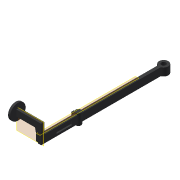
# Autodesk Inventor part: lock
Saved by Autodesk Inventor 2022 Beta2 (Build 260130000, 130) ContinuousBuild 0
## iProperties
Shininess: 64.0
Length Units: 11269
Angle Units: 11279
Time Units: 11290
Mass Units: 11286
Length Display Precision: 3
Angle Display Precision: 2
Created: 2002-04-26
Part Number: lock
Document SubType Name: Modeling
Designer: Administrator
Density: 1 g/cm^3
Material: Generic
Appearance: Generic
Density: 0.0
Volumn: 0.0
Area: 0.0
PropertySet Name: Model Information
Control State: 0
Master: False
Checked Out: False
Author: Administrator
Autodesk Inventor part; units mm, degrees
ref_plane "YZ Plane" through (0, 0, 0) normal (1, 0, 0) x (0, 1, 0)
ref_plane "XZ Plane" through (0, 0, 0) normal (0, 1, 0) x (-1, 0, 0)
ref_plane "XY Plane" through (0, 0, 0) normal (0, 0, 1) x (1, 0, 0)
sketch "Sketch1" plane through (0, 0, 0) normal (0, 0, 1) x (1, 0, 0)
  line L0 (-33.82, 21.26) -> (-13.5, 21.26)
  line L1 (-13.5, 21.26) -> (-13.5, 6.02)
  line L2 (-13.5, 6.02) -> (-16.04, 6.02)
  line L3 (-16.04, 6.02) -> (-18.58, 16.18)
  line L4 (-18.58, 16.18) -> (-33.82, 16.18)
  line L5 (-33.82, 16.18) -> (-33.82, 21.26)
  dimension "d0" = 20.32
  dimension "d1" = 15.24
  dimension "d2" = 5.08
  dimension "d3" = 2.54
  dimension "d4" = 15.24
  constraints: 12 end point, 3 parallel, 1 horizontal, 1 perpendicular
  measures "d0" distance of L0.start L0.end
  measures "d1" distance of L0.end L1.end
  measures "d2" distance of L4.end L0.start
  measures "d3" distance of L1.end L2.end
  measures "d4" distance of L3.end L4.end
extrude "Extrusion1" add sketch "Sketch1" along normal blind 2.54
ref_plane "Work Plane1" through (0, 0, 1.27) normal (0, 0, 1) x (1, 0, 0)
sketch "Sketch2" plane through (0, 0, 1.27) normal (0, 0, 1) x (1, 0, 0)
  line L0 (-33.82, 18.974) -> (-36.36, 18.974)
  arc A0 (-36.36, 18.974) -> (-35.5534, 12.624) centre (-10.96, 18.974) ccw
  line L1 (-35.5534, 12.624) -> (-33.82, 12.624)
  line L2 (-33.82, 12.624) -> (-33.82, 18.974)
  line L3 (-33.82, 16.18) -> (-33.82, 21.26) projected
  line L4 (-33.82, 21.26) -> (-13.5, 21.26) projected
  dimension "d8" = 2.54
  dimension "d9" = 6.35
  dimension "d10" = 25.4
  dimension "d11" = 2.286
  constraints: 6 end point, 2 point on circle, 1 centre point, 1 collinear, 1 horizontal, 1 parallel, 1 perpendicular, 1 point on line
  measures "d8" distance of L0.start L0.end
  measures "d9" distance from line of L0 L1.end
  measures "d10" radius of A0
  measures "d11" distance between parallel lines of L0 L4
revolve "Revolution1" add sketch "Sketch2" angle 360 about axis through (-33.82, 18.974, 1.27) along (-1, 0, 0)
sketch "Sketch3" plane through (0, 0, 1.27) normal (0, 0, 1) x (1, 0, 0)
  line L0 (-16.04, 6.02) -> (-18.58, 6.02)
  line L1 (-18.58, 6.02) -> (-18.58, 18.72)
  line L2 (-18.58, 18.72) -> (-16.04, 18.72)
  line L3 (-16.04, 18.72) -> (-16.04, 6.02)
  line L4 (-13.5, 6.02) -> (-16.04, 6.02) projected
  dimension "d13" = 12.7
  dimension "d14" = 2.54
  constraints: 8 end point, 2 parallel, 1 collinear, 1 horizontal, 1 perpendicular
  measures "d13" distance of L0.end L1.end
  measures "d14" distance of L0.start L0.end
extrude "Extrusion2" add sketch "Sketch3" along normal mid plane 1.016
sketch "Sketch4" plane through (-13.5, 6.02, 0) normal (1, 0, 0) x (0, 0, -1)
  line L0 (-2.54, 15.24) -> (-2.54, 0) projected
  line L1 (0, 15.24) -> (-2.54, 15.24) projected
  line L2 (-2.54, 0) -> (99.06, 0)
  line L3 (-2.54, 6.35) -> (99.06, 6.35)
  line L4 (99.06, 6.35) -> (99.06, 0)
  dimension "d17" = 6.35
  dimension "d18" = 101.6
  constraints: 6 end point, 2 parallel, 1 perpendicular, 1 point on line
  measures "d17" distance of L3.end L2.end
  measures "d18" distance of L0.end L2.end
extrude "Extrusion3" add sketch "Sketch4" against normal blind 2.54
ref_plane "Work Plane2" through (-13.5, 13.64, 0) normal (0, 1, 0) x (1, 0, 0)
sketch "Sketch5" plane through (-13.5, 13.64, 0) normal (0, 1, 0) x (1, 0, 0)
  circle A0 centre (-1.27, 29.21) radius 2.286
  line L0 (0, 99.06) -> (0, 0) projected
  line L1 (-20.32, -2.54) -> (0, -2.54) projected
  dimension "d22" = 4.572
  dimension "d23" = 1.27
  dimension "d24" = 31.75
  constraints: 1 centre point
  measures "d22" diameter of A0
  measures "d23" distance from line of L0 A0.centre
  measures "d24" distance from line of A0.centre L1
extrude "Extrusion4" add sketch "Sketch5" against normal blind 8.89
sketch "Sketch6" plane through (-16.04, 12.37, 0) normal (0, 1, 0) x (1, 0, 0)
  arc A0 (0, 27.3092) -> (2.54, 27.3092) centre (1.27, 29.21) ccw projected
  line L0 (0, 27.3092) -> (0, 0) projected
  line L1 (2.54, 27.3092) -> (2.54, 0) projected
  line L2 (1.27, 29.21) -> (-2.54, 29.21)
  line L3 (-2.54, 29.21) -> (-2.54, 27.178)
  line L4 (-2.54, 27.178) -> (1.27, 27.178)
  line L5 (1.27, 27.178) -> (1.27, 29.21)
  line L6 (-2.54, -1.778) -> (-2.54, -0.762) projected
  dimension "d27" = 2.032
  constraints: 8 end point, 3 perpendicular, 1 collinear, 1 parallel
  measures "d27" distance of L2.end L3.end
extrude "Extrusion5" add sketch "Sketch6" against normal up to surface (6.35 mm away)
sketch "Sketch7" plane through (-16.04, 6.02, -99.06) normal (0, -1, 0) x (1, 0, 0)
  line L0 (0, 67.9492) -> (0, 0) projected
  line L1 (2.54, 67.9492) -> (2.54, 0) projected
  circle A0 centre (1.27, 0) radius 3.81
  circle A1 centre (1.27, 0) radius 1.27 construction
  arc A2 (2.54, 71.7508) -> (-1.016, 69.85) centre (1.27, 69.85) ccw projected
  dimension "d31" = 7.62
  dimension "d42" = 69.85
  constraints: 2 centre point, 2 tangent, 1 concentric
  measures "d31" diameter of A0
  measures "d42" distance of A0.centre A2.centre
extrude "Extrusion6" add sketch "Sketch7" against normal up to surface (6.35 mm away)
sketch "Sketch8" plane through (-14.77, 6.02, -29.21) normal (0, -1, 0) x (1, 0, 0)
  arc A0 (-1.27, -66.2579) -> (1.27, -66.2579) centre (0, -69.85) ccw projected
hole "Hole1" at (-14.77, 6.02, -99.06) direction (0, 1, 0) diameter 3.81 end through all
sketch "Sketch9" plane through (-13.5, 6.02, 2.54) normal (1, 0, 0) x (0, 0, -1)
  line L0 (29.8492, 6.35) -> (2.54, 6.35) projected
  line L1 (0, 0) -> (29.8492, 0) projected
  circle A0 centre (14.8195, 3.175) radius 3.175 construction
  line L2 (0, 15.24) -> (0, 0) projected
  line L3 (12.7, 4.699) -> (25.4, 4.699)
  line L4 (25.4, 4.699) -> (25.4, 1.651)
  line L5 (25.4, 1.651) -> (12.7, 1.651)
  line L6 (12.7, 1.651) -> (12.7, 4.699)
  circle A1 centre (14.8195, 3.175) radius 1.524 construction
  dimension "d46" = 12.7
  dimension "d47" = 12.7
  dimension "d48" = 3.048
  constraints: 8 end point, 4 tangent, 2 centre point, 2 parallel, 1 coincident, 1 horizontal, 1 perpendicular
  measures "d46" distance of L3.start L3.end
  measures "d47" distance between parallel lines of L2 L6
  measures "d48" distance of L3.end L4.end
extrude "Extrusion7" cut sketch "Sketch9" against normal blind 1.27
body "Solid1"
